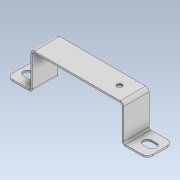
# Autodesk Inventor part: Скоба БП1
Saved by Autodesk Inventor 2021.2 (Build 252289000, 289)
## iProperties
Created: 2022-11-30
Part Number: Скоба БП1
Material: Типовые
Document SubType Name: ЛистМат
Designer: Voodoo
Mass: 1.75231 g
Surface Area: 38.2715 cm^2
Volume: 1.75231 cm^3
Density: 1 g/cm^3
Sheet Metal Rule: По умолчанию_мм
Appearance: По умолчанию
Flat Pattern Width: 1.5 cm
Flat Pattern Length: 12.2048 cm
Flat Pattern Area: 18.3072 cm^2
Sheet Metal Width: 15,000 мм
Sheet Metal Length: 122,048 мм
Sheet Metal Area: 1830,717 мм^2
Author: Voodoo
Autodesk Inventor part; units mm, degrees
ref_plane "YZ Plane" through (0, 0, 0) normal (1, 0, 0) x (0, 1, 0)
ref_plane "XZ Plane" through (0, 0, 0) normal (0, 1, 0) x (-1, 0, 0)
ref_plane "XY Plane" through (0, 0, 0) normal (0, 0, 1) x (1, 0, 0)
sketch "Эскиз1" plane through (0, 0, 0) normal (0, 0, 1) x (1, 0, 0)
  line L0 (0, 0) -> (53, 0) construction
  line L1 (53, 0) -> (53, 21)
  line L2 (53, 21) -> (0, 21)
  line L3 (0, 21) -> (0, 0)
  line L4 (0, 0) -> (-15, 0)
  line L5 (53, 0) -> (68, 0)
  dimension "d0" = 53
  dimension "d1" = 21
  dimension "d2" = 15
  dimension "d3" = 15
  measures "d0" distance of L1.end L2.end
  measures "d1" distance between parallel lines of L0 L2
  measures "d2" distance of L0.start L4.end
  measures "d3" distance of L0.end L5.end
contour flange "Фланец по контуру1" sketch "Эскиз1" thickness 1 bend radius 1 width 15 along (0, 0, 1) mid plane no both sides no wall seen from (-7.5, 0, 0) lies toward (0, 1, 0) curves L4 L3 L2 L1 L5
bend "Сгиб1"
corner "УглСтык1"
sketch "Эскиз2" plane through (68, 1, 15) normal (0, 1, 0) x (1, 0, 0)
  line L0 (-70, 15) -> (-70, 0) projected
  line L1 (-83, 15) -> (-70, 15) projected
  line L2 (-83, 0) -> (-83, 15) projected
  line L3 (-70, 0) -> (-83, 0) projected
  line L4 (-13, 15) -> (-13, 0) projected
  line L5 (0, 0) -> (-13, 0) projected
  line L6 (0, 15) -> (0, 0) projected
  line L7 (-13, 15) -> (0, 15) projected
  line L8 (-7.5, 7.5) -> (-4.5, 7.5) construction
  line L9 (-7.5, 5) -> (-4.5, 5)
  line L10 (-4.5, 10) -> (-7.5, 10)
  arc A0 (-7.5, 10) -> (-7.5, 5) centre (-7.5, 7.5) ccw
  arc A1 (-4.5, 5) -> (-4.5, 10) centre (-4.5, 7.5) ccw
  line L11 (-78.5, 7.5) -> (-75.5, 7.5) construction
  line L12 (-78.5, 5) -> (-75.5, 5)
  line L13 (-75.5, 10) -> (-78.5, 10)
  arc A2 (-78.5, 10) -> (-78.5, 5) centre (-78.5, 7.5) ccw
  arc A3 (-75.5, 5) -> (-75.5, 10) centre (-75.5, 7.5) ccw
  point P0 (-68, 15)
  point P1 (-6, 7.5)
  point P2 (-77, 7.5)
  point P3 (-83, 7.5)
  point P4 (0, 7.5)
  dimension "d15" = 3
  dimension "d16" = 5
  dimension "d17" = 3
  dimension "d18" = 5
  dimension "d19" = 6
  dimension "d20" = 6
  constraints: 16 end point, 8 point on circle, 8 tangent, 4 centre point, 4 midpoint, 2 horizontal, 2 horizontal alignment, 2 parallel
  measures "d15" distance of L8.start L8.end
  measures "d16" diameter of A1
  measures "d17" distance of L11.start L11.end
  measures "d18" diameter of A3
  measures "d19" distance from line of L6 point (-6, 7.5)
  measures "d20" distance from line of L2 point (-77, 7.5)
extrude "Вырез1" cut sketch "Эскиз2" against normal blind 1 contours A0 L10 A1 L9 | A2 L13 A3 L12
fillet "УглСкругление1" radius 3 4 edges at (-15, 0.5, 15) (-15, 0.5, 0) (68, 0.5, 15) (68, 0.5, 0)
sketch "Эскиз3" plane through (1, 22, 0) normal (0, 1, 0) x (1, 0, 0)
  line L0 (51, 0) -> (51, -15) projected
  line L1 (0, 0) -> (51, 0) projected
  line L2 (0, 0) -> (0, -15) projected
  line L3 (51, -15) -> (0, -15) projected
  circle A0 centre (43, -7.5) radius 1.5
  point P0 (-1, 0)
  point P1 (51, -7.5)
  dimension "d24" = 3
  dimension "d25" = 8
  constraints: 1 centre point, 1 horizontal alignment, 1 midpoint
  measures "d24" diameter of A0
  measures "d25" distance from line of A0.centre L0
extrude "Вырез2" cut sketch "Эскиз3" against normal blind 1 contours A0
equation "\"d21\" = Толщина"
equation "\"d26\" = Толщина"
equation "\"d4\" = Толщина"
equation "\"d5\" = Ширина_просечки"
equation "\"d6\" = Глубина_просечки"
equation "\"d7\" = Мин_остаток"
equation "\"d8\" = Радиус_перехода"
equation "\"d10\" = Радиус_гибки"
equation "\"d12\" = Размер_просечки"
equation "\"d13\" = Размер_зазора"
equation "\"d14\" = Радиус_Якоби"
equation "\"Радиус_гибки\" = Толщина"
equation "\"Ширина_просечки\" = Толщина"
equation "\"Глубина_просечки\" = 0.5 * Толщина"
equation "\"Размер_просечки\" = 4 * Толщина"
equation "\"Мин_остаток\" = 2 * Толщина"
equation "\"Радиус_перехода\" = Радиус_гибки"
equation "\"Радиус_Якоби\" = Радиус_гибки"
equation "\"Размер_зазора\" = Толщина"
equation "\"Толщина\" = 1"
